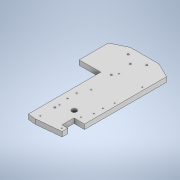
# Autodesk Inventor part: montageplaatje
Saved by Autodesk Inventor 2021 (Build 250183000, 183)
## iProperties
Created: 2022-11-09
Part Number: montageplaatje
Material: Generic
Document SubType Name: Modeling
Designer: marti
Density: 1 g/cm^3
Appearance: Default
Author: marti
Autodesk Inventor part; units mm, degrees
ref_plane "YZ Plane" through (0, 0, 0) normal (1, 0, 0) x (0, 1, 0)
ref_plane "XZ Plane" through (0, 0, 0) normal (0, 1, 0) x (-1, 0, 0)
ref_plane "XY Plane" through (0, 0, 0) normal (0, 0, 1) x (1, 0, 0)
sketch "Sketch1" plane through (0, 0, 0) normal (0, 1, 0) x (-1, 0, 0)
  line L0 (19.5, -173) -> (0, -173) construction
  line L1 (0, -173) -> (-19.5, -173) construction
  line L2 (61, -173) -> (61, 35)
  line L3 (0, 0) -> (0, -173) construction
  line L4 (0, -188) -> (30, -188)
  line L5 (61, -173) -> (30, -188)
  line L6 (61, 35) -> (0, 41)
  line L7 (-61, -173) -> (-61, 35)
  line L8 (0, -188) -> (-30, -188)
  line L9 (-61, -173) -> (-30, -188)
  line L10 (-61, 35) -> (0, 41)
  point P0 (0, -118)
  point P1 (0, -158)
  dimension "d0" = 118
  dimension "d1" = 40
  dimension "d2" = 19.5
  dimension "d3" = 15
  dimension "d4" = 61
  dimension "d6" = 15
  dimension "d7" = 35
  dimension "d8" = 41
  dimension "d11" = 30
  constraints: 22 end point, 4 vertical alignment, 3 symmetric about line, 2 collinear, 2 horizontal, 2 vertical, 1 coincident, 1 horizontal alignment
  measures "d0" distance of point (0, 0) point (0, -118)
  measures "d1" distance of point (0, -118) point (0, -158)
  measures "d2" horizontal distance of point (0, -158) L0.start
  measures "d3" vertical distance of point (0, -158) L0.start
  measures "d4" distance between parallel lines of L3 L2
  measures "d6" distance from line of L0.start L4
  measures "d7" vertical distance of L2.end L3.start
  measures "d8" distance of L3.start L6.end
  measures "d11" horizontal distance of L0.end L4.end
extrude "uitlijn plaatje" add sketch "Sketch1" along normal blind 10
hole "Hole1" at (-19.5, 0, -173) at (19.5, 0, -173) at (0, 0, 0) at (0, 0, -118) at (0, 0, -158) direction (0, 1, 0) diameter 3.4 end through all clearance for "Hex Head Cap Screw ISO 24017" size "M3" standard "ISO"
sketch "batterij uitsnijding" plane through (0, 10, 0) normal (0, 1, 0) x (1, 0, 0)
  line L0 (-61, -35) -> (0, -41) projected
  line L1 (-16, -39.4262) -> (-16, 112)
  line L2 (-16, 112) -> (-61, 112)
  line L3 (-61, 173) -> (-61, -35) projected
  point P0 (0, 0)
  dimension "d21" = 45
  dimension "d22" = 112
  constraints: 4 end point, 1 perpendicular, 1 point on line, 1 vertical
  measures "d21" distance between parallel lines of L3 L1
  measures "d22" distance from line of point (0, 0) L2
extrude "Extrusion2" cut sketch "batterij uitsnijding" against normal blind 10
sketch "Sketch3" plane through (0, 10, 0) normal (0, 1, 0) x (1, 0, 0)
  circle A0 centre (25.75, 14.75) radius 5
  point P0 (0, 0)
  dimension "d26" = 14.75
  dimension "d27" = 25.75
  dimension "d28" = 10
  constraints: 1 centre point
  measures "d26" vertical distance of A0.centre point (0, 0)
  measures "d27" horizontal distance of A0.centre point (0, 0)
  measures "d28" diameter of A0
extrude "Extrusion3" cut sketch "Sketch3" against normal blind 10
sketch "Sketch4" plane through (0, 10, 0) normal (0, 1, 0) x (1, 0, 0)
  line L0 (56.6557, 151.7192) -> (-9.4519, 151.7192)
  line L1 (-9.4519, 151.7192) -> (-9.4519, 66.7192)
  line L2 (-9.4519, 66.7192) -> (56.6557, 66.7192)
  line L3 (56.6557, 66.7192) -> (56.6557, 151.7192)
  point P0 (0, 0)
  point P1 (0, -30.4368)
  point P2 (0, 9.5632)
  point P3 (45, -30.4368)
  point P4 (45, 9.5632)
  point P5 (51.8228, 48.7167)
  point P6 (51.8228, 29.7167)
  point P7 (-3.1772, 48.7167)
  point P8 (-3.1772, 29.7167)
  point P9 (5.7892, 70.2192)
  point P10 (54.7892, 70.2192)
  point P11 (54.7892, 128.2192)
  point P12 (5.7892, 128.2192)
  dimension "d31" = 40
  dimension "d32" = 45
  dimension "d33" = 19
  dimension "d34" = 55
  dimension "d35" = 58
  dimension "d36" = 49
  dimension "d37" = 55
  dimension "d38" = 19
  dimension "d39" = 85
  dimension "d40" = 3.5
  constraints: 8 end point, 6 vertical alignment, 4 horizontal alignment, 2 parallel, 1 horizontal, 1 perpendicular
  measures "d31" distance of point (0, 9.563) point (0, -30.437)
  measures "d32" distance of point (45, -30.437) point (0, -30.437)
  measures "d33" distance of point (51.823, 29.717) point (51.823, 48.717)
  measures "d34" distance of point (51.823, 48.717) point (-3.177, 48.717)
  measures "d35" distance of point (5.789, 128.219) point (5.789, 70.219)
  measures "d36" distance of point (54.789, 70.219) point (5.789, 70.219)
  measures "d37" distance of point (51.823, 29.717) point (-3.177, 29.717)
  measures "d38" distance of point (-3.177, 48.717) point (-3.177, 29.717)
  measures "d39" distance of L0.end L1.end
  measures "d40" distance from line of L2 point (5.789, 70.219)
hole "Hole2" at (0, 10, 30.4368) at (0, 10, -9.5632) at (45, 10, 30.4368) at (45, 10, -9.5632) at (51.8228, 10, -48.7167) at (51.8228, 10, -29.7167) at (-3.1772, 10, -48.7167) at (-3.1772, 10, -29.7167) at (5.7892, 10, -70.2192) at (54.7892, 10, -70.2192) at (54.7892, 10, -128.2192) at (5.7892, 10, -128.2192) direction (0, -1, 0) diameter 2.2 end through all
sketch "Sketch5" plane through (0, 10, 0) normal (0, 1, 0) x (1, 0, 0)
  line L0 (0, -41) -> (61, -35) projected
  line L1 (51, -35.9836) -> (51, -23.9836)
  line L2 (51, -23.9836) -> (39, -23.9836)
  line L3 (39, -23.9836) -> (39, 1.0164)
  line L4 (39, 1.0164) -> (54.3101, 1.0164)
  line L5 (54.3101, 1.0164) -> (61, 1.0164)
  line L6 (61, -35) -> (61, 173) projected
  point P0 (0, 0)
  dimension "d48" = 25
  dimension "d49" = 12
  dimension "d50" = 10
  dimension "d51" = 12
  constraints: 10 end point, 3 perpendicular, 3 point on line, 1 vertical
  measures "d48" distance of L2.end L3.end
  measures "d49" distance of L1.start L1.end
  measures "d50" distance between parallel lines of L6 L1
  measures "d51" distance of L1.end L2.end
extrude "Extrusion4" cut sketch "Sketch5" against normal blind 10
body "Solid1"
